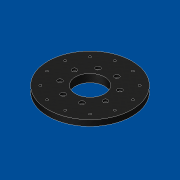
# Autodesk Inventor part: 201-
Saved by Autodesk Inventor 2018 (Build 220112000, 112)
## iProperties
Created: 2020-01-12
Part Number: 201-
Material: Generic
Document SubType Name: Modeling
Designer: Bunny320
Density: 1 g/cm^3
Appearance: Diamond plate - Dark Gray
Author: Bunny320
## iProperties of the stored document 105-flange adapter_3DPrint.ipt
Created: 2020-05-11
Part Number: 105-flange adapter_3DPrint
Material: Generic
Document SubType Name: Modeling
Designer: Bunny320
Density: 1 g/cm^3
Appearance: Default
Author: Bunny320
Autodesk Inventor part; units mm, degrees
ref_plane "YZ Plane" through (0, 0, 0) normal (1, 0, 0) x (0, 1, 0)
ref_plane "XZ Plane" through (0, 0, 0) normal (0, 1, 0) x (-1, 0, 0)
ref_plane "XY Plane" through (0, 0, 0) normal (0, 0, 1) x (1, 0, 0)
sketch "Sketch1" plane through (0, 0, 0) normal (0, 0, 1) x (1, 0, 0)
  circle A0 centre (0, 0) radius 35
  point P0 (0, 35)
  point P1 (0, -35)
  dimension "d0" = 70
  constraints: 2 point on circle, 1 centre point, 1 coincident
  measures "d0" diameter of A0
extrude "Extrusion1" add sketch "Sketch1" along normal blind 3
sketch "Sketch3" plane through (0, 0, 3) normal (0, 0, 1) x (1, 0, 0)
  circle A0 centre (0, 0) radius 57.5
  dimension "d8" = 115
  constraints: 1 centre point, 1 coincident
  measures "d8" diameter of A0
extrude "Extrusion3" add sketch "Sketch3" along normal blind 8
sketch "Sketch7" plane through (0, 0, 11) normal (0, 0, 1) x (1, 0, 0)
  line L0 (-15, 25.9808) -> (0, 0)
  line L1 (0, 80.5) -> (0, -80.5) projected
  dimension "d25" = 30
  dimension "d26" = 30
  constraints: 2 end point
  measures "d25" distance of L0.start L0.end
  measures "d26" angle of L1 L0
hole "Hole2" at (-15, 25.9808, 11) direction (0, 0, -1) diameter 3.4 end through all counterbore diameter 6.5 counterbore depth 3.4 clearance for "Socket Head Cap Screw DIN EN ISO 4762" size "M3" standard "DIN"
pattern_circular "Circular Pattern1" count 8 over 360 about axis through (0, 0, -10) along (0, 0, 1) of "Hole2"
sketch "Sketch12" plane through (0, 0, 11) normal (0, 0, 1) x (1, 0, 0)
  line L0 (-12.4233, 46.3644) -> (0, 0)
  line L1 (0, 80.5) -> (0, -80.5) projected
  dimension "d77" = 15
  dimension "d78" = 48
  constraints: 2 end point
  measures "d77" angle of L1 L0
  measures "d78" distance of L0.start L0.end
hole "Hole6" at (-12.4233, 46.3644, 11) direction (0, 0, -1) diameter 3.2 end through all
pattern_circular "Circular Pattern2" count 12 over 360 about axis through (0, 0, -10) along (0, 0, 1) of "Hole6"
sketch "Sketch8" plane through (0, 0, 11) normal (0, 0, 1) x (1, 0, 0)
  circle A0 centre (0, 0) radius 20
  dimension "d89" = 40
  constraints: 2 coincident, 1 centre point
  measures "d89" diameter of A0
extrude "Extrusion4" cut sketch "Sketch8" against normal through all
equation "\"d79\" = M3_adjustable"
equation "\"bearing_61807_inner\" = 35"
equation "\"bearing_61807_outer\" = 47.1"
equation "\"bearing_61814_outer\" = 90.1"
equation "\"M3_adjustable\" = 3.2"
body "Solid1"
